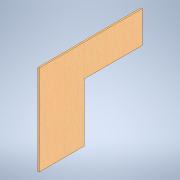
# Autodesk Inventor part: Side Part
Saved by Autodesk Inventor 2022.2 (Build 262287000, 287)
## iProperties
Created: 2022-02-23
Part Number: Side Part
Material: Pine, Southern
Document SubType Name: Modeling
Designer: PRASHANTH
Density: 0.570257 g/cm^3
Appearance: Yellow Pine - Stained Dark Medium Gloss
Author: PRASHANTH
Autodesk Inventor part; units mm, degrees
ref_plane "YZ Plane" through (0, 0, 0) normal (1, 0, 0) x (0, 1, 0)
ref_plane "XZ Plane" through (0, 0, 0) normal (0, 1, 0) x (-1, 0, 0)
ref_plane "XY Plane" through (0, 0, 0) normal (0, 0, 1) x (1, 0, 0)
sketch "Sketch1" plane through (0, 0, 0) normal (1, 0, 0) x (0, 1, 0)
  line L0 (-157.5, -42.5) -> (62.5, -42.5)
  line L1 (62.5, -42.5) -> (62.5, -262.5)
  line L2 (62.5, -262.5) -> (157.5, -262.5)
  line L3 (-157.5, -42.5) -> (-157.5, 127.5)
  line L4 (182.5, 127.5) -> (-157.5, 127.5)
  line L5 (62.5, -262.5) -> (182.5, -262.5)
  line L6 (182.5, -262.5) -> (182.5, 127.5)
  point P0 (0, 0)
  point P1 (157.5, 127.5)
  dimension "d8" = 170
  dimension "d9" = 120
  constraints: 14 end point, 2 perpendicular, 2 point on line, 2 vertical, 1 horizontal
  measures "d8" distance of L0.start L3.end
  measures "d9" distance of L1.end L5.end
extrude "Extrusion1" add sketch "Sketch1" along normal blind 5
body "Solid1"
